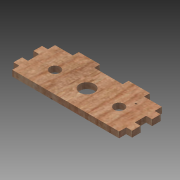
# Autodesk Inventor part: holder_plate
Saved by Autodesk Inventor 2015 (Build 190159000, 159)
## iProperties
Created: 2013-12-24
Part Number: holder_plate
Material: Wood (Birch)
Document SubType Name: Modeling
Designer: aoki
Density: 1 g/cm^3
Appearance: Birch - Natural Polished
d21: 100.000 mm
d22: 40.000 mm
d23: 5.500 mm
d24: 0.00 deg
d52: 60.000 mm
d53: 9.600 mm
d122: 14.000 mm
Author: aoki
Autodesk Inventor part; units mm, degrees
ref_plane "YZ Plane" through (0, 0, 0) normal (1, 0, 0) x (0, 1, 0)
ref_plane "XZ Plane" through (0, 0, 0) normal (0, 1, 0) x (-1, 0, 0)
ref_plane "XY Plane" through (0, 0, 0) normal (0, 0, 1) x (1, 0, 0)
sketch "Block1" plane through (0, 0, 0) normal (0, 0, 1) x (1, 0, 0)
  line L0 (-37.5521, 20) -> (-37.5521, 24)
  line L1 (-37.5521, 24) -> (-17.5521, 24)
  line L2 (-17.5521, 24) -> (-17.5521, 20)
  line L3 (-37.4196, 20) -> (-17.5521, 20)
  line L4 (17.5521, 24) -> (17.5521, 20)
  line L5 (37.5521, 20) -> (37.5521, 24)
  line L6 (37.5521, 24) -> (17.5521, 24)
  line L7 (37.4196, 20) -> (17.5521, 20)
  point P0 (0, 21.8462)
  dimension "d140" = 20
  dimension "d141" = 4
  measures "d140" distance of L0.end L1.end
  measures "d141" distance of L0.start L0.end
sketch "Block2" plane through (0, 0, 0) normal (0, 0, 1) x (1, 0, 0)
  line L0 (-33.5533, 20.22) -> (-33.5533, 29.22)
  line L1 (-33.5533, 29.22) -> (-13.1133, 29.22)
  line L2 (-13.1133, 29.22) -> (-13.1133, 20.22)
  line L3 (-13.1133, 20.22) -> (13.1133, 20.22)
  line L4 (13.1133, 20.22) -> (13.1133, 29.22)
  line L5 (13.1133, 29.22) -> (33.5533, 29.22)
  line L6 (33.5533, 29.22) -> (33.5533, 20.22)
  line L7 (33.5533, 20.22) -> (50.22, 20.22)
  line L8 (50.22, 20.22) -> (50.22, 13.5533)
  line L9 (50.22, 13.5533) -> (59.22, 13.5533)
  line L10 (59.22, 13.5533) -> (59.22, 5.1133)
  line L11 (59.22, 5.1133) -> (50.22, 5.1133)
  line L12 (50.22, 5.1133) -> (50.22, -5.1133)
  line L13 (50.22, -5.1133) -> (59.22, -5.1133)
  line L14 (59.22, -5.1133) -> (59.22, -13.5533)
  line L15 (59.22, -13.5533) -> (50.22, -13.5533)
  line L16 (50.22, -13.5533) -> (50.22, -20.22)
  line L17 (50.22, -20.22) -> (-50.22, -20.22)
  line L18 (-50.22, -20.22) -> (-50.22, -13.5533)
  line L19 (-50.22, -13.5533) -> (-59.22, -13.5533)
  line L20 (-59.22, -13.5533) -> (-59.22, -5.1133)
  line L21 (-59.22, -5.1133) -> (-50.22, -5.1133)
  line L22 (-50.22, -5.1133) -> (-50.22, 5.1133)
  line L23 (-50.22, 5.1133) -> (-59.22, 5.1133)
  line L24 (-59.22, 5.1133) -> (-59.22, 13.5533)
  line L25 (-59.22, 13.5533) -> (-50.22, 13.5533)
  line L26 (-50.22, 13.5533) -> (-50.22, 20.22)
  line L27 (-50.22, 20.22) -> (-33.5533, 20.22)
  circle A0 centre (-30, 0) radius 4.72
  circle A1 centre (0, 0) radius 4.72
  circle A2 centre (30, 0) radius 4.72
  point P0 (0, 6.592)
sketch "Block3" plane through (0, 0, 0) normal (0, 0, 1) x (1, 0, 0)
  line L0 (-33.4333, 29.1) -> (-13.2333, 29.1)
  line L1 (-13.2333, 29.1) -> (-13.2333, 20.1)
  line L2 (-13.2333, 20.1) -> (13.2333, 20.1)
  line L3 (13.2333, 20.1) -> (13.2333, 29.1)
  line L4 (13.2333, 29.1) -> (33.4333, 29.1)
  line L5 (33.4333, 29.1) -> (33.4333, 20.1)
  line L6 (33.4333, 20.1) -> (50.1, 20.1)
  line L7 (50.1, 20.1) -> (50.1, 13.4333)
  line L8 (50.1, 13.4333) -> (59.1, 13.4333)
  line L9 (59.1, 13.4333) -> (59.1, 5.2333)
  line L10 (59.1, 5.2333) -> (50.1, 5.2333)
  line L11 (50.1, 5.2333) -> (50.1, -5.2333)
  line L12 (50.1, -5.2333) -> (59.1, -5.2333)
  line L13 (59.1, -5.2333) -> (59.1, -13.4333)
  line L14 (59.1, -13.4333) -> (50.1, -13.4333)
  line L15 (50.1, -13.4333) -> (50.1, -20.1)
  line L16 (50.1, -20.1) -> (-50.1, -20.1)
  line L17 (-50.1, -20.1) -> (-50.1, -13.4333)
  line L18 (-50.1, -13.4333) -> (-59.1, -13.4333)
  line L19 (-59.1, -13.4333) -> (-59.1, -5.2333)
  line L20 (-59.1, -5.2333) -> (-50.1, -5.2333)
  line L21 (-50.1, -5.2333) -> (-50.1, 5.2333)
  line L22 (-50.1, 5.2333) -> (-59.1, 5.2333)
  line L23 (-59.1, 5.2333) -> (-59.1, 13.4333)
  line L24 (-59.1, 13.4333) -> (-50.1, 13.4333)
  line L25 (-50.1, 13.4333) -> (-50.1, 20.1)
  line L26 (-50.1, 20.1) -> (-33.4333, 20.1)
  line L27 (-33.4333, 20.1) -> (-33.4333, 29.1)
  circle A0 centre (-30, 0) radius 5.6
  circle A1 centre (0, 0) radius 7.1
  circle A2 centre (30, 0) radius 5.6
  point P0 (0, 6.56)
sketch "Block4" plane through (0, 0, 0) normal (0, 0, 1) x (1, 0, 0)
  line L0 (-33.5333, 29.2) -> (-13.1333, 29.2)
  line L1 (-13.1333, 29.2) -> (-13.1333, 20.2)
  line L2 (-13.1333, 20.2) -> (13.1333, 20.2)
  line L3 (13.1333, 20.2) -> (13.1333, 29.2)
  line L4 (13.1333, 29.2) -> (33.5333, 29.2)
  line L5 (33.5333, 29.2) -> (33.5333, 20.2)
  line L6 (33.5333, 20.2) -> (50.2, 20.2)
  line L7 (50.2, 20.2) -> (50.2, 13.5333)
  line L8 (50.2, 13.5333) -> (59.2, 13.5333)
  line L9 (59.2, 13.5333) -> (59.2, 5.1333)
  line L10 (59.2, 5.1333) -> (50.2, 5.1333)
  line L11 (50.2, 5.1333) -> (50.2, -5.1333)
  line L12 (50.2, -5.1333) -> (59.2, -5.1333)
  line L13 (59.2, -5.1333) -> (59.2, -13.5333)
  line L14 (59.2, -13.5333) -> (50.2, -13.5333)
  line L15 (50.2, -13.5333) -> (50.2, -20.2)
  line L16 (50.2, -20.2) -> (-50.2, -20.2)
  line L17 (-50.2, -20.2) -> (-50.2, -13.5333)
  line L18 (-50.2, -13.5333) -> (-59.2, -13.5333)
  line L19 (-59.2, -13.5333) -> (-59.2, -5.1333)
  line L20 (-59.2, -5.1333) -> (-50.2, -5.1333)
  line L21 (-50.2, -5.1333) -> (-50.2, 5.1333)
  line L22 (-50.2, 5.1333) -> (-59.2, 5.1333)
  line L23 (-59.2, 5.1333) -> (-59.2, 13.5333)
  line L24 (-59.2, 13.5333) -> (-50.2, 13.5333)
  line L25 (-50.2, 13.5333) -> (-50.2, 20.2)
  line L26 (-50.2, 20.2) -> (-33.5333, 20.2)
  line L27 (-33.5333, 20.2) -> (-33.5333, 29.2)
  circle A0 centre (-30, 0) radius 5.7
  circle A1 centre (0, 0) radius 7.2
  circle A2 centre (30, 0) radius 5.7
  point P0 (0, 6.5867)
sketch "Block5" plane through (0, 0, 0) normal (0, 0, 1) x (1, 0, 0)
  line L0 (13.2333, 29.1) -> (33.4333, 29.1)
  line L1 (33.4333, 29.1) -> (33.4333, 20.1)
  line L2 (33.4333, 20.1) -> (50.1, 20.1)
  line L3 (50.1, 20.1) -> (50.1, 13.4333)
  line L4 (50.1, 13.4333) -> (59.1, 13.4333)
  line L5 (59.1, 13.4333) -> (59.1, 5.2333)
  line L6 (59.1, 5.2333) -> (50.1, 5.2333)
  line L7 (50.1, 5.2333) -> (50.1, -5.2333)
  line L8 (50.1, -5.2333) -> (59.1, -5.2333)
  line L9 (59.1, -5.2333) -> (59.1, -13.4333)
  line L10 (59.1, -13.4333) -> (50.1, -13.4333)
  line L11 (50.1, -13.4333) -> (50.1, -20.1)
  line L12 (50.1, -20.1) -> (-50.1, -20.1)
  line L13 (-50.1, -20.1) -> (-50.1, -13.4333)
  line L14 (-50.1, -13.4333) -> (-59.1, -13.4333)
  line L15 (-59.1, -13.4333) -> (-59.1, -5.2333)
  line L16 (-59.1, -5.2333) -> (-50.1, -5.2333)
  line L17 (-50.1, -5.2333) -> (-50.1, 5.2333)
  line L18 (-50.1, 5.2333) -> (-59.1, 5.2333)
  line L19 (-59.1, 5.2333) -> (-59.1, 13.4333)
  line L20 (-59.1, 13.4333) -> (-50.1, 13.4333)
  line L21 (-50.1, 13.4333) -> (-50.1, 20.1)
  line L22 (-50.1, 20.1) -> (-33.4333, 20.1)
  line L23 (-33.4333, 20.1) -> (-33.4333, 29.1)
  line L24 (-33.4333, 29.1) -> (-13.2333, 29.1)
  line L25 (-13.2333, 29.1) -> (-13.2333, 20.1)
  line L26 (-13.2333, 20.1) -> (13.2333, 20.1)
  line L27 (13.2333, 20.1) -> (13.2333, 29.1)
  circle A0 centre (-30, 0) radius 5.6
  circle A1 centre (0, 0) radius 7.1
  circle A2 centre (30, 0) radius 5.6
  point P0 (0, 6.56)
sketch "Block6" plane through (0, 0, 0) normal (0, 0, 1) x (1, 0, 0)
  line L0 (-33.4133, 25.58) -> (-13.2533, 25.58)
  line L1 (-13.2533, 25.58) -> (-13.2533, 20.08)
  line L2 (-13.2533, 20.08) -> (13.2533, 20.08)
  line L3 (13.2533, 20.08) -> (13.2533, 25.58)
  line L4 (13.2533, 25.58) -> (33.4133, 25.58)
  line L5 (33.4133, 25.58) -> (33.4133, 20.08)
  line L6 (33.4133, 20.08) -> (50.08, 20.08)
  line L7 (50.08, 20.08) -> (50.08, 13.4133)
  line L8 (50.08, 13.4133) -> (55.58, 13.4133)
  line L9 (55.58, 13.4133) -> (55.58, 5.2533)
  line L10 (55.58, 5.2533) -> (50.08, 5.2533)
  line L11 (50.08, 5.2533) -> (50.08, -5.2533)
  line L12 (50.08, -5.2533) -> (55.58, -5.2533)
  line L13 (55.58, -5.2533) -> (55.58, -13.4133)
  line L14 (55.58, -13.4133) -> (50.08, -13.4133)
  line L15 (50.08, -13.4133) -> (50.08, -20.08)
  line L16 (50.08, -20.08) -> (-50.08, -20.08)
  line L17 (-50.08, -20.08) -> (-50.08, -13.4133)
  line L18 (-50.08, -13.4133) -> (-55.58, -13.4133)
  line L19 (-55.58, -13.4133) -> (-55.58, -5.2533)
  line L20 (-55.58, -5.2533) -> (-50.08, -5.2533)
  line L21 (-50.08, -5.2533) -> (-50.08, 5.2533)
  line L22 (-50.08, 5.2533) -> (-55.58, 5.2533)
  line L23 (-55.58, 5.2533) -> (-55.58, 13.4133)
  line L24 (-55.58, 13.4133) -> (-50.08, 13.4133)
  line L25 (-50.08, 13.4133) -> (-50.08, 20.08)
  line L26 (-50.08, 20.08) -> (-33.4133, 20.08)
  line L27 (-33.4133, 20.08) -> (-33.4133, 25.58)
  circle A0 centre (-30, 0) radius 5.58
  circle A1 centre (0, 0) radius 7.08
  circle A2 centre (30, 0) radius 5.58
  point P0 (0, 6.088)
sketch "Block7" plane through (0, 0, 0) normal (0, 0, 1) x (1, 0, 0)
  line L0 (-33.4133, 25.58) -> (-13.2533, 25.58)
  line L1 (-13.2533, 25.58) -> (-13.2533, 20.08)
  line L2 (-13.2533, 20.08) -> (13.2533, 20.08)
  line L3 (13.2533, 20.08) -> (13.2533, 25.58)
  line L4 (13.2533, 25.58) -> (33.4133, 25.58)
  line L5 (33.4133, 25.58) -> (33.4133, 20.08)
  line L6 (33.4133, 20.08) -> (50.08, 20.08)
  line L7 (50.08, 20.08) -> (50.08, 13.4133)
  line L8 (50.08, 13.4133) -> (55.58, 13.4133)
  line L9 (55.58, 13.4133) -> (55.58, 5.2533)
  line L10 (55.58, 5.2533) -> (50.08, 5.2533)
  line L11 (50.08, 5.2533) -> (50.08, -5.2533)
  line L12 (50.08, -5.2533) -> (55.58, -5.2533)
  line L13 (55.58, -5.2533) -> (55.58, -13.4133)
  line L14 (55.58, -13.4133) -> (50.08, -13.4133)
  line L15 (50.08, -13.4133) -> (50.08, -20.08)
  line L16 (50.08, -20.08) -> (-50.08, -20.08)
  line L17 (-50.08, -20.08) -> (-50.08, -13.4133)
  line L18 (-50.08, -13.4133) -> (-55.58, -13.4133)
  line L19 (-55.58, -13.4133) -> (-55.58, -5.2533)
  line L20 (-55.58, -5.2533) -> (-50.08, -5.2533)
  line L21 (-50.08, -5.2533) -> (-50.08, 5.2533)
  line L22 (-50.08, 5.2533) -> (-55.58, 5.2533)
  line L23 (-55.58, 5.2533) -> (-55.58, 13.4133)
  line L24 (-55.58, 13.4133) -> (-50.08, 13.4133)
  line L25 (-50.08, 13.4133) -> (-50.08, 20.08)
  line L26 (-50.08, 20.08) -> (-33.4133, 20.08)
  line L27 (-33.4133, 20.08) -> (-33.4133, 25.58)
  circle A0 centre (-30, 0) radius 4.88
  circle A1 centre (0, 0) radius 7.08
  circle A2 centre (30, 0) radius 4.88
  point P0 (0, 6.088)
sketch "Sketch10" plane through (0, 0, 0) normal (0, 0, 1) x (1, 0, 0)
  line L0 (50, -20) -> (-50, -20)
  line L1 (-50, -20) -> (-50, 20)
  line L2 (-50, 20) -> (50, 20)
  line L3 (50, 20) -> (50, -20)
  line L4 (50, -20) -> (-50, 20) construction
  line L5 (-50, -20) -> (50, 20) construction
  point P0 (0, 0)
  dimension "d21" = 100
  dimension "d22" = 40
  constraints: 12 end point, 2 midpoint, 2 parallel, 1 horizontal, 1 perpendicular
  measures "d21" distance of L1.end L2.end
  measures "d22" distance of L0.end L1.end
extrude "Extrusion2" add sketch "Sketch10" against normal blind 5.5
sketch "Sketch16" plane through (0, 0, -5.5) normal (0, 0, -1) x (-1, 0, 0)
  line L0 (0, -30.0399) -> (0, 39.5395) projected
  point P0 (0, 0)
  point P1 (-30, 0)
  point P2 (30, 0)
  dimension "d52" = 60
  constraints: 1 symmetric about line
  measures "d52" distance of point (30, 0) point (-30, 0)
hole "Hole5" at (30, 0, -5.5) at (-30, 0, -5.5) direction (0, 0, 1) diameter 9.6 end through all
sketch "Sketch17" plane through (0, 0, -5.5) normal (0, 0, -1) x (-1, 0, 0)
  point P0 (0, 0)
  point P1 (0, 0)
  constraints: 1 coincident
hole "Hole14" at (0, 0, -5.5) direction (0, 0, 1) diameter 14 end through all
sketch "Sketch34" plane through (0, 0, 0) normal (0, 0, 1) x (1, 0, 0)
  line L0 (-50, 20) -> (50, 20) projected
  line L1 (-50, -20) -> (-50, 20) projected
  line L2 (-30, 20) -> (-10, 20)
  line L3 (0, -30.0399) -> (0, 39.5395) projected
  line L4 (-234.7041, 0) -> (108.0673, 0) projected
  line L5 (-30, 20) -> (-30, 25.5)
  line L6 (-10, 20) -> (-10, 25.5)
  line L7 (-10, 25.5) -> (-30, 25.5)
  line L8 (30, 20) -> (10, 20)
  line L9 (30, 20) -> (30, 25.5)
  line L10 (10, 20) -> (10, 25.5)
  line L11 (10, 25.5) -> (30, 25.5)
  line L12 (-50, 13.3333) -> (-55.5, 13.3333)
  line L13 (-55.5, 13.3333) -> (-55.5, 5.3333)
  line L14 (-55.5, 5.3333) -> (-50, 5.3333)
  line L15 (-50, 13.3333) -> (-50, 5.3333)
  line L16 (50, 13.3333) -> (55.5, 13.3333)
  line L17 (55.5, 13.3333) -> (55.5, 5.3333)
  line L18 (55.5, 5.3333) -> (50, 5.3333)
  line L19 (50, 13.3333) -> (50, 5.3333)
  line L20 (-50, -13.3333) -> (-55.5, -13.3333)
  line L21 (-55.5, -13.3333) -> (-55.5, -5.3333)
  line L22 (-55.5, -5.3333) -> (-50, -5.3333)
  line L23 (-50, -13.3333) -> (-50, -5.3333)
  line L24 (50, -13.3333) -> (50, -5.3333)
  line L25 (55.5, -13.3333) -> (55.5, -5.3333)
  line L26 (55.5, -5.3333) -> (50, -5.3333)
  line L27 (50, -13.3333) -> (55.5, -13.3333)
  dimension "d131" = 20
  dimension "d132" = 5.5
  dimension "d133" = 5.5
  dimension "d134" = 8
  dimension "d135" = 6.6667
  constraints: 48 end point, 16 symmetric about line, 4 perpendicular, 4 point on line, 2 collinear, 2 parallel
  measures "d131" distance of L6.end L5.end
  measures "d132" distance of L2.start L5.end
  measures "d133" distance of L12.start L12.end
  measures "d134" distance of L12.end L13.end
  measures "d135" distance between parallel lines of L0 L12
extrude "Extrusion4" add sketch "Sketch34" against normal blind 5.5 contours L1 L20 L21 L22 | L1 L14 L13 L12 | L16 L17 L18 L19 | L24 L26 L25 L27
sketch "Sketch35" plane through (0, 0, 0) normal (0, 0, 1) x (1, 0, 0)
  line L0 (-50, 20) -> (50, 20) projected
  line L1 (-50, 13.3333) -> (-50, 20) projected
  line L2 (0, -30.0399) -> (0, 39.5395) projected
  line L3 (-33.3333, 20) -> (-13.3333, 20)
  line L4 (-13.3333, 20) -> (-13.3333, 25.5)
  line L5 (-13.3333, 25.5) -> (-33.3333, 25.5)
  line L6 (-33.3333, 25.5) -> (-33.3333, 20)
  line L7 (33.3333, 20) -> (13.3333, 20)
  line L8 (13.3333, 20) -> (13.3333, 25.5)
  line L9 (13.3333, 25.5) -> (33.3333, 25.5)
  line L10 (33.3333, 25.5) -> (33.3333, 20)
  dimension "d142" = 16.6667
  dimension "d143" = 20
  dimension "d144" = 5.5
  constraints: 16 end point, 4 symmetric about line, 2 parallel, 1 horizontal, 1 perpendicular, 1 point on line
  measures "d142" distance between parallel lines of L1 L6
  measures "d143" distance of L4.end L5.end
  measures "d144" distance of L3.end L4.end
extrude "Extrusion5" add sketch "Sketch35" against normal blind 5.5
equation "\"d140\" = 0.2 * d21"
equation "\"d141\" = At"
equation "\"d23\" = Wt"
equation "\"d131\" = 0.2 * d21"
equation "\"d132\" = Wt"
equation "\"d133\" = Wt"
equation "\"d134\" = 0.2 * d22"
equation "\"d135\" = 0.166667 * d22"
equation "\"d138\" = Wt"
equation "\"d142\" = 0.166667 * d21"
equation "\"d143\" = 0.2 * d21"
equation "\"d144\" = Wt"
equation "\"d145\" = Wt"
equation "\"At\" = 4"
equation "\"Wt\" = 5.5"
body "Solid2"
